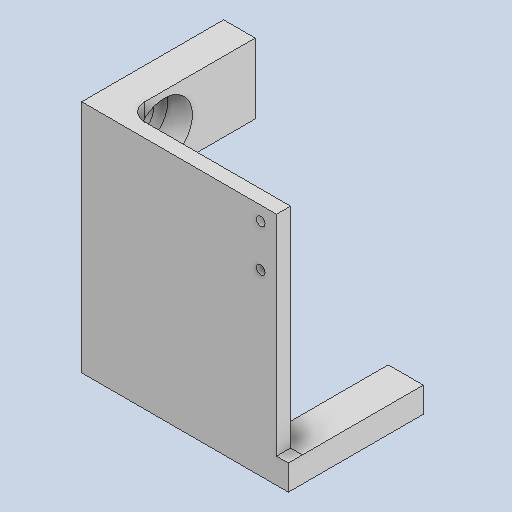
# Autodesk Inventor part: Soporte mecanismo
Saved by Autodesk Inventor 2023 (Build 270158000, 158)
## iProperties
Created: 2022-12-03
Part Number: Soporte mecanismo
Material: Genérico
Document SubType Name: Modeling
Designer: sergi
Density: 1 g/cm^3
Appearance: Valor por defecto
Author: sergi
Autodesk Inventor part; units mm, degrees
ref_plane "YZ Plane" through (0, 0, 0) normal (1, 0, 0) x (0, 1, 0)
sketch "Boceto1" plane through (0, 0, 0) normal (0, 0, 1) x (1, 0, 0)
  line L0 (25, 19.2857) -> (25, 3.2857) projected
  line L1 (20, 19.2857) -> (20, 3.2857) projected
  line L2 (-26.6, 19.2857) -> (-26.6, 3.2857) projected
  line L3 (-21.6, 19.2857) -> (-21.6, 3.2857) projected
  line L4 (25, 19.2857) -> (20, 19.2857)
  line L5 (25, 3.2857) -> (20, 3.2857)
  line L6 (-21.6, 3.2857) -> (-26.6, 3.2857)
  line L7 (-21.6, 19.2857) -> (-26.6, 19.2857)
  line L8 (-28.6, 1.2857) -> (-28.6, 21.2857)
  line L9 (-28.6, 21.2857) -> (-19.6, 21.2857)
  line L10 (-19.6, 21.2857) -> (-19.6, 1.2857)
  line L11 (-19.6, 1.2857) -> (-28.6, 1.2857)
  line L12 (18, 1.2857) -> (18, 21.2857)
  line L13 (18, 21.2857) -> (27, 21.2857)
  line L14 (27, 21.2857) -> (27, 1.2857)
  line L15 (27, 1.2857) -> (18, 1.2857)
  line L16 (-26.7, 3.1857) -> (-26.7, 19.3857)
  line L17 (-26.7, 19.3857) -> (-21.5, 19.3857)
  line L18 (-21.5, 19.3857) -> (-21.5, 3.1857)
  line L19 (-21.5, 3.1857) -> (-26.7, 3.1857)
  line L20 (19.9, 3.1857) -> (19.9, 19.3857)
  line L21 (19.9, 19.3857) -> (25.1, 19.3857)
  line L22 (25.1, 19.3857) -> (25.1, 3.1857)
  line L23 (25.1, 3.1857) -> (19.9, 3.1857)
  point P0 (0, 0)
  dimension "d0" = 2
  dimension "d1" = 2
  dimension "d2" = 0.1
  dimension "d3" = 0.1
  constraints: 40 end point, 4 horizontal, 12 other
  measures "d0" distance between parallel lines of L2 L8
  measures "d1" distance between parallel lines of L1 L12
  measures "d2" distance between parallel lines of L2 L16
  measures "d3" distance between parallel lines of L1 L20
extrude "Extrusión1" add sketch "Boceto1" along normal blind 40.5 contours L7 L3 L6 L2 | L8 L9 L10 L11 | L16 L17 L18 L19
sketch "Boceto2" plane through (-19.6, 1.2857, 0) normal (1, 0, 0) x (0, 0, -1)
  circle A0 centre (-26, 10) radius 8 projected
  point P0 (0, -1.2857)
hole "Agujero1" at (-19.6, 11.2857, 26) direction (-1, 0, 0) diameter 8 end through all both
sketch "Boceto3" plane through (-19.6, 1.2857, 0) normal (1, 0, 0) x (0, 0, -1)
  circle A0 centre (-26, 10) radius 8 projected
  point P0 (0, -1.2857)
hole "Agujero2" at (-19.6, 11.2857, 26) direction (-1, 0, 0) diameter 16.2 depth 7
sketch "Boceto5" plane through (0, 0, 40.5) normal (0, 0, 1) x (1, 0, 0)
  line L0 (27, 21.2857) -> (-28.6, 21.2857)
  line L1 (-28.6, 21.2857) -> (-28.6, -45.7143)
  line L2 (-28.6, -45.7143) -> (27, -45.7143)
  line L3 (27, -45.7143) -> (27, 21.2857)
  point P0 (0, 0)
  dimension "d27" = 55.6
  dimension "d28" = 67
  constraints: 8 end point, 2 parallel, 1 horizontal, 1 perpendicular
  measures "d27" distance of L2.end L1.end
  measures "d28" distance of L1.end L0.end
extrude "Extrusión2" add sketch "Boceto5" against normal blind 4
sketch "Boceto6" plane through (0, 0, 36.5) normal (0, 0, -1) x (-1, 0, 0)
  circle A0 centre (0, -16.5) radius 8 projected
  point P0 (0, 0)
hole "Agujero4" at (0, -16.5, 36.5) direction (0, 0, 1) diameter 16.2 depth 2
sketch "Boceto7" plane through (0, 0, 36.5) normal (0, 0, -1) x (-1, 0, 0)
  line L0 (19.6, 21.2857) -> (-27, 21.2857) projected
  line L1 (-27, 21.2857) -> (-18, 21.2857)
  line L2 (-18, 21.2857) -> (-18, 1.2857)
  line L3 (-18, 1.2857) -> (-27, 1.2857)
  line L4 (-27, 1.2857) -> (-27, 21.2857)
  line L5 (-22.5, 1.2857) -> (-22.5, 21.2857)
  line L6 (-22.5, 21.2857) -> (-22.5, 17.2857)
  circle A0 centre (-22.5, 17.2857) radius 1.25
  line L7 (-22.5, 1.2857) -> (-22.5, 5.2857)
  circle A1 centre (-22.5, 5.2857) radius 1.25
  point P0 (0, 0)
  dimension "d38" = 9
  dimension "d39" = 4
  dimension "d40" = 2.5
  dimension "d41" = 4
  dimension "d42" = 2.5
  constraints: 14 end point, 2 centre point, 2 coincident, 2 midpoint, 2 parallel, 2 point on line, 1 horizontal, 1 perpendicular
  measures "d38" distance of L2.end L3.end
  measures "d39" distance of L5.end L6.end
  measures "d40" diameter of A0
  measures "d41" distance of L5.start L7.end
  measures "d42" diameter of A1
hole "Agujero5" at (22.5, 5.2857, 36.5) at (22.5, 17.2857, 36.5) direction (0, 0, 1) diameter 2.5 depth 4
sketch "Boceto9" plane through (0, 0, 0) normal (0, 0, -1) x (-1, 0, 0)
  line L0 (19.6, 21.2857) -> (28.6, 21.2857) projected
  line L1 (24.1, 21.2857) -> (24.1, 17.2857)
  line L2 (24.1, 17.2857) -> (24.1, 9.2857)
  circle A0 centre (24.1, 17.2857) radius 1.25
  circle A1 centre (24.1, 9.2857) radius 1.25
  point P0 (0, 0)
  dimension "d50" = 4
  dimension "d51" = 8
  dimension "d52" = 2.5
  dimension "d53" = 2.5
  constraints: 4 end point, 2 centre point, 2 coincident, 1 midpoint, 1 point on line, 1 vertical
  measures "d50" distance of L1.start L1.end
  measures "d51" distance of L1.end L2.end
  measures "d52" diameter of A0
  measures "d53" diameter of A1
hole "Agujero6" at (-24.1, 17.2857, 0) at (-24.1, 9.2857, 0) direction (0, 0, 1) diameter 2.5 depth 10
sketch "Boceto10" plane through (0, 0, 36.5) normal (0, 0, -1) x (-1, 0, 0)
  line L0 (28.6, -45.7143) -> (-27, -45.7143) projected
  line L1 (-27, -45.7143) -> (-19, -45.7143)
  line L2 (-27, -45.7143) -> (28.6, -45.7143) projected
  line L3 (28.6, -45.7143) -> (20.6, -45.7143)
  line L4 (20.6, -45.7143) -> (20.6, -36.7143)
  line L5 (20.6, -36.7143) -> (28.6, -36.7143)
  line L6 (28.6, -36.7143) -> (28.6, -45.7143)
  circle A0 centre (-25.3717, -42.5) radius 1.25
  line L7 (-30.3717, -46.5) -> (-30.3717, -38.5)
  line L8 (-20.3717, -38.5) -> (-30.3717, -38.5)
  line L9 (-20.3717, -44.5) -> (-20.3717, -38.5)
  line L10 (-20.3717, -44.5) -> (-20.3717, -46.5)
  circle A1 centre (25.3717, -42.5) radius 1.25
  line L11 (20.3717, -38.5) -> (20.3717, -44.5)
  line L12 (-30.3717, -38.5) -> (-20.3717, -38.5)
  line L13 (-20.3717, -38.5) -> (-20.3717, -45.7143)
  line L14 (-20.3717, -45.7143) -> (-30.3717, -45.7143)
  line L15 (-30.3717, -45.7143) -> (-30.3717, -38.5)
  point P0 (0, 0)
  point P1 (-20.3717, -45.7143)
  dimension "d75" = 8
  dimension "d76" = 9
  constraints: 28 end point, 4 horizontal, 4 parallel, 4 vertical, 2 centre point, 2 perpendicular, 1 point on line, 11 other
  measures "d75" distance of L4.end L5.end
  measures "d76" distance of L3.end L4.end
ref_plane "Plano de trabajo1" through (-48.5, -48.5, 0) normal (0, 0, 1) x (1, 0, 0)
ref_plane "Plano de trabajo2" through (20.3717, -44.5, 2.0001) normal (0, 0, 1) x (1, 0, 0)
extrude "Extrusión3" add sketch "Boceto10" along normal up to surface (34.4999 mm away) contours L0 L4 L5 L6 | L0 L14 L7 L8 L9 L10 | A0 | A1
fillet "Empalme1" radius 5 4 edges at (-24.1, 1.2857, 36.5) (-19.6, 11.2857, 36.5) (-20.6, -41.2143, 36.5) (-24.6, -36.7143, 36.5)
sketch "Boceto12" plane through (27, -45.7143, 40.5) normal (1, 0, 0) x (0, 0, -1)
  line L0 (4, 7.2143) -> (4, 0) projected
  line L1 (4, 0) -> (0, 0)
  line L2 (0, 0) -> (0, 7.214)
  line L3 (0, 7.214) -> (4, 7.214)
  line L4 (4, 7.214) -> (4, 0)
  point P0 (40.5, 45.7143)
  dimension "d79" = 4
  dimension "d80" = 7.214
  constraints: 8 end point, 2 parallel, 1 horizontal, 1 perpendicular
  measures "d79" distance of L2.end L3.end
  measures "d80" distance of L1.end L2.end
extrude "Extrusión4" add sketch "Boceto12" along normal up to surface (3.3717 mm away)
sketch "Boceto13" plane through (30.3717, -45.7143, 2.0001) normal (0, 0, -1) x (-1, 0, 0)
  circle A0 centre (5, 3.2143) radius 1.25 projected
  circle A1 centre (55.7434, 3.2143) radius 1.25 projected
  point P0 (30.3717, 45.7143)
hole "Agujero8" at (25.3717, -42.5, 2.0001) at (-25.3717, -42.5, 2.0001) direction (0, 0, 1) diameter 2.5 depth 8
